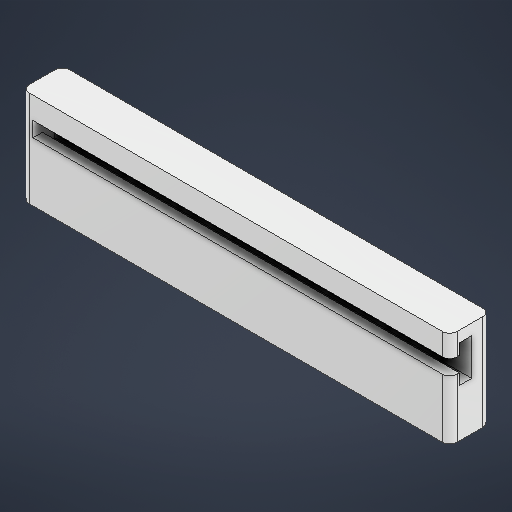
# Autodesk Inventor part: module-slot
Saved by Autodesk Inventor 2025.4 (Build 294407000, 407)
## iProperties
Created: 2025-12-31
Part Number: module-slot
Material: PC/ABS Plastic
Document SubType Name: Modeling
Designer: sam
Density: 1.1 g/cm^3
Appearance: Smooth - White
Author: sam
Autodesk Inventor part; units mm, degrees
ref_plane "YZ Plane" through (0, 0, 0) normal (1, 0, 0) x (0, 1, 0)
ref_plane "XZ Plane" through (0, 0, 0) normal (0, 1, 0) x (-1, 0, 0)
ref_plane "XY Plane" through (0, 0, 0) normal (0, 0, 1) x (1, 0, 0)
sketch "Sketch1" plane through (0, 0, 0) normal (0, 0, 1) x (1, 0, 0)
  line L0 (58.4, 13.1) -> (-58.4, 13.1)
  line L1 (-58.4, 13.1) -> (-58.4, -13.1)
  line L2 (-58.4, -13.1) -> (58.4, -13.1)
  line L3 (58.4, -13.1) -> (58.4, 13.1)
  line L4 (58.4, 13.1) -> (-58.4, -13.1) construction
  line L5 (-58.4, 13.1) -> (58.4, -13.1) construction
  point P0 (0, 0)
  dimension "d0" = 116.8
  dimension "d1" = 26.2
  constraints: 12 end point, 2 midpoint, 2 parallel, 1 horizontal, 1 perpendicular
  measures "d0" distance of L2.end L1.end
  measures "d1" distance of L1.end L0.end
extrude "Extrusion1" add sketch "Sketch1" along normal blind 11
sketch "Sketch2" plane through (58.4, -13.1, 0) normal (1, 0, 0) x (0, 0, -1)
  line L0 (0, 0) -> (0, 26.2) projected
  line L1 (0, 26.2) -> (-11, 26.2) projected
  line L2 (-11, 0) -> (-11, 26.2) projected
  line L3 (0, 0) -> (-11, 0) projected
  line L4 (-11, 26.2) -> (-11, 0) projected
  line L5 (-11, 26.2) -> (-5, 26.2)
  line L6 (-5, 26.2) -> (-5, 23.2)
  line L7 (-5, 23.2) -> (-11, 23.2)
  line L8 (-11, 23.2) -> (-11, 26.2)
  line L9 (-11, 23.2) -> (-8.4, 23.2)
  line L10 (-8.4, 23.2) -> (-8.4, 20.2)
  line L11 (-8.4, 20.2) -> (-11, 20.2)
  line L12 (-11, 20.2) -> (-11, 23.2)
  line L13 (-11, 26.2) -> (-5, 26.2)
  line L14 (-5, 26.2) -> (-5, 10.1)
  line L15 (-5, 10.1) -> (-11, 10.1)
  line L16 (-11, 10.1) -> (-11, 26.2)
  line L17 (-11, 10.1) -> (-5, 10.1)
  line L18 (-5, 10.1) -> (-5, 13.1)
  line L19 (-5, 13.1) -> (-11, 13.1)
  line L20 (-11, 13.1) -> (-11, 10.1)
  line L21 (-11, 13.1) -> (-8.4, 13.1)
  line L22 (-8.4, 13.1) -> (-8.4, 16.1)
  line L23 (-8.4, 16.1) -> (-11, 16.1)
  line L24 (-11, 16.1) -> (-11, 13.1)
  point P0 (0, 13.1)
  point P1 (-11, 16.1)
  point P2 (-11, 20.2)
  dimension "d4" = 6
  dimension "d5" = 3
  dimension "d6" = 2.6
  dimension "d7" = 3
  dimension "d8" = 16.1
  dimension "d9" = 3
  dimension "d10" = 2.6
  dimension "d11" = 3
  constraints: 40 end point, 10 parallel, 5 horizontal, 5 perpendicular, 1 point on line
  measures "d4" distance of L6.end L7.end
  measures "d5" distance of L5.end L6.end
  measures "d6" distance of L10.end L11.end
  measures "d7" distance of L9.end L10.end
  measures "d8" distance of L13.end L14.end
  measures "d9" distance of L18.end L17.end
  measures "d10" distance of L23.end L22.end
  measures "d11" distance of L22.end L21.end
extrude "Extrusion2" cut sketch "Sketch2" against normal blind 113.8 contours L14 L19 L22 L23 L2 L11 L10 L7
fillet "Fillet1" radius 2 5 edges at (58.4, 10.1, 11) (58.4, -5.05, 11) (-58.4, 0, 11) (58.4, 0, 0) (-58.4, 0, 0)
sketch "Sketch4" plane through (-56.4, -13.1, 0) normal (0, -1, 0) x (1, 0, 0)
  arc A0 (-2, 2) -> (0, 0) centre (0, 2) ccw projected
  line L0 (0, 0) -> (112.8, 0) projected
  arc A1 (112.8, 0) -> (114.8, 2) centre (112.8, 2) ccw projected
  line L1 (114.8, 2) -> (114.8, 9) projected
  arc A2 (114.8, 9) -> (112.8, 11) centre (112.8, 9) ccw projected
  line L2 (0, 11) -> (112.8, 11) projected
  arc A3 (0, 11) -> (-2, 9) centre (0, 9) ccw projected
  line L3 (-2, 2) -> (-2, 9) projected
  circle A4 centre (104.8, 5.5) radius 4.1
  circle A5 centre (97.8, 5.5) radius 2.15
  line L4 (97.8, 7.65) -> (101.3089, 7.65)
  line L5 (97.8, 3.35) -> (101.3089, 3.35)
  circle A6 centre (15, 5.5) radius 4.1
  circle A7 centre (8, 5.5) radius 2.15
  line L6 (8, 3.35) -> (11.5089, 3.35)
  line L7 (8, 7.65) -> (11.5089, 7.65)
  point P0 (56.4, 0)
  point P1 (114.8, 5.5)
  point P2 (12.2407, 8.5325)
  point P3 (8.4381, 3.3951)
  point P4 (11.1965, 3.9692)
  point P5 (-2, 5.5)
  dimension "d19" = 8.2
  dimension "d20" = 4.3
  dimension "d21" = 7
  dimension "d22" = 0
  dimension "d23" = 10
  dimension "d24" = 8.2
  dimension "d25" = 4.3
  dimension "d26" = 7
  dimension "d27" = 10
  dimension "d28" = 0
  dimension "d40" = 0
  constraints: 11 point on circle, 8 end point, 4 centre point, 2 midpoint, 2 parallel, 2 tangent, 1 horizontal
  measures "d19" diameter of A4
  measures "d20" diameter of A5
  measures "d21" distance of A4.centre A5.centre
  measures "d22" vertical distance of point (114.8, 5.5) A4.centre
  measures "d23" distance from line of L1 A4.centre
  measures "d24" diameter of A6
  measures "d25" diameter of A7
  measures "d26" distance of A6.centre A7.centre
  measures "d27" distance from line of L3 A7.centre
  measures "d28" vertical distance of point (-2, 5.5) A6.centre
  measures "d40" vertical distance of A6.centre A7.centre
extrude "Extrusion4" cut sketch "Sketch4" against normal blind 5.2 contours A4 | A4 L5 A5 L4 | A5 | A6 | A6 L6 A7 L7 | A7
sketch "Sketch5" plane through (-56.4, -13.1, 0) normal (0, -1, 0) x (1, 0, 0)
  arc A0 (8, 7.65) -> (8, 3.35) centre (8, 5.5) ccw projected
  arc A1 (11.5089, 3.35) -> (11.5089, 7.65) centre (15, 5.5) ccw projected
  arc A2 (97.8, 7.65) -> (97.8, 3.35) centre (97.8, 5.5) ccw projected
  line L0 (97.8, 7.65) -> (101.3089, 7.65) projected
  arc A3 (101.3089, 3.35) -> (101.3089, 7.65) centre (104.8, 5.5) ccw projected
  line L1 (101.3089, 3.35) -> (97.8, 3.35) projected
  arc A4 (-2, 2) -> (0, 0) centre (0, 2) ccw projected
  line L2 (0, 0) -> (112.8, 0) projected
  arc A5 (112.8, 0) -> (114.8, 2) centre (112.8, 2) ccw projected
  line L3 (114.8, 2) -> (114.8, 9) projected
  arc A6 (114.8, 9) -> (112.8, 11) centre (112.8, 9) ccw projected
  line L4 (0, 11) -> (112.8, 11) projected
  arc A7 (0, 11) -> (-2, 9) centre (0, 9) ccw projected
  line L5 (-2, 2) -> (-2, 9) projected
  circle A8 centre (8, 5.5) radius 4.1
  line L6 (8, 9.6) -> (15, 9.6)
  line L7 (8, 1.4) -> (15, 1.4)
  arc A9 (11.5089, 3.35) -> (11.5089, 7.65) centre (15, 5.5) ccw projected
  circle A10 centre (97.8, 5.5) radius 4.1
  line L8 (97.8, 9.6) -> (104.8, 9.6)
  line L9 (104.8, 1.4) -> (97.8, 1.4)
  line L10 (8, 7.65) -> (11.5089, 7.65) projected
  line L11 (11.5089, 3.35) -> (8, 3.35) projected
  arc A11 (8, 7.65) -> (8, 3.35) centre (8, 5.5) ccw projected
  point P0 (56.4, 0)
  point P1 (19.1, 5.5)
  point P2 (19.1, 5.5)
  point P3 (5.85, 5.5)
  point P4 (95.65, 5.5)
  point P5 (12.4867, 2.2607)
  point P6 (12.4867, 8.7393)
  point P7 (96.275, 2.2698)
  point P8 (96.275, 8.7302)
  point P9 (5.85, 5.5)
  point P10 (101.2911, 7.65)
  point P11 (101.2911, 3.35)
  point P12 (11.4911, 3.35)
  point P13 (11.4911, 7.65)
  dimension "d32" = 8.2
  dimension "d33" = 0
  dimension "d35" = 8.2
  dimension "d36" = 0
  dimension "d42" = 0
  dimension "d43" = 0
  constraints: 11 point on circle, 8 end point, 4 tangent, 2 centre point, 1 horizontal
  measures "d32" diameter of A8
  measures "d33" distance of A0.centre A8.centre
  measures "d35" diameter of A10
  measures "d36" distance of A2.centre A10.centre
  measures "d42" distance of A8.centre A0.centre
  measures "d43" distance of A10.centre A2.centre
extrude "Extrusion5" cut sketch "Sketch5" along normal blind 3.2 from surface at -5.2 contours L10 A8 L11 A0 | A0 L11 A8 L10 | A8 L6 A1 L10 | L11 A1 L7 A8 | L0 A10 L1 A2 | A2 L1 A10 L0 | A10 L8 A3 L0 | L1 A3 L9 A10
body "Solid1"
